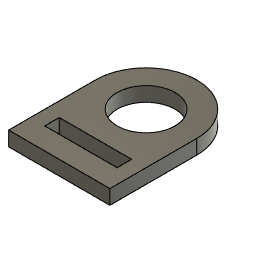
ex1 (Autodesk Fusion 360 design; units mm, degrees)
Autodesk Fusion 360 part; units mm, degrees
sketch "Sketch1" plane through (0, 0, 0) normal (0, 1, 0) x (1, 0, 0)
  line L0 (0, 0) -> (70, 0)
  line L1 (0, 0) -> (0, 60)
  line L2 (70, 0) -> (70, 60)
  circle A0 centre (35, 60) radius 20
  line L3 (60, 15) -> (60, 25)
  line L4 (60, 25) -> (10, 25)
  line L5 (10, 25) -> (10, 15)
  line L6 (10, 15) -> (60, 15)
  arc A1 (70, 60) -> (0, 60) centre (35, 60) ccw
  dimension "d1" = 70
  dimension "d2" = 60
  dimension "d3" = 40
  dimension "d4" = 50
  dimension "d5" = 10
  constraint coincident L0.start L1.start
  constraint horizontal L0
  constraint perpendicular L0 L1
  constraint perpendicular L0 L2
  constraint perpendicular L2 L4
  constraint perpendicular L4 L5
  constraint perpendicular L3 L6
  constraint coincident A0.centre A1.centre
  measures "d1" distance of L0.start L0.end
  measures "d2" distance of L0.start L1.end
  measures "d3" diameter of A0
  measures "d4" distance of L3.end L4.end
  measures "d5" distance of L4.end L5.end
extrude "Extrude1" add sketch "Sketch1" along normal blind 10
